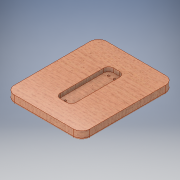
# Autodesk Inventor part: Stand
Saved by Autodesk Inventor 2017 (Build 210142000, 142)
## iProperties
Created: 2018-11-02
Part Number: Stand
Material: Wood (Oak)
Document SubType Name: Modeling
Designer: 623516
Density: 0.76 g/cm^3
Appearance: White Oak - Natural Medium Gloss
Author: 623516
Autodesk Inventor part; units mm, degrees
ref_plane "YZ Plane" through (0, 0, 0) normal (1, 0, 0) x (0, 1, 0)
ref_plane "XZ Plane" through (0, 0, 0) normal (0, 1, 0) x (-1, 0, 0)
ref_plane "XY Plane" through (0, 0, 0) normal (0, 0, 1) x (1, 0, 0)
sketch "Sketch1" plane through (0, 0, 0) normal (0, 1, 0) x (-1, 0, 0)
  line L0 (0, 0) -> (180, 0)
  line L1 (180, 0) -> (180, -220)
  line L2 (180, -220) -> (0, -220)
  line L3 (0, -220) -> (0, 0)
  line L4 (90, 0) -> (90, -220) construction
  line L5 (90, -110) -> (90, -161.5) construction
  line L6 (90, -110) -> (90, -58.5) construction
  line L7 (90, -161.5) -> (83, -161.5) construction
  line L8 (83, -161.5) -> (83, -193.1088) construction
  circle A0 centre (83, -161.5) radius 2.5
  line L9 (90, -161.5) -> (97, -161.5) construction
  circle A1 centre (97, -161.5) radius 2.5
  line L10 (90, -58.5) -> (83, -58.5) construction
  line L11 (83, -58.5) -> (83, 21.6306) construction
  circle A2 centre (83, -58.5) radius 2.5
  line L12 (90, -58.5) -> (97, -58.5) construction
  circle A3 centre (97, -58.5) radius 2.5 construction
  circle A4 centre (97, -58.5) radius 2.5
  dimension "d0" = 180
  dimension "d1" = 220
  dimension "d2" = 51.5
  dimension "d3" = 51.5
  dimension "d4" = 7
  dimension "d5" = 5
  dimension "d6" = 7
  dimension "d7" = 5
  dimension "d8" = 7
  dimension "d9" = 5
  dimension "d10" = 7
  dimension "d11" = 5
  dimension "d12" = 5
  constraints: 26 end point, 5 centre point, 5 coincident, 5 perpendicular, 3 horizontal, 3 midpoint, 2 parallel, 2 point on line
  measures "d0" distance of L1.end L2.end
  measures "d1" distance of L0.end L1.end
  measures "d2" distance of L5.start L5.end
  measures "d3" distance of L5.start L6.end
  measures "d4" distance of L5.end L7.end
  measures "d5" diameter of A0
  measures "d6" distance of L5.end L9.end
  measures "d7" diameter of A1
  measures "d8" distance of L6.end L10.end
  measures "d9" diameter of A2
  measures "d10" distance of L6.end L12.end
  measures "d11" diameter of A3
  measures "d12" diameter of A4
extrude "Extrusion1" add sketch "Sketch1" along normal blind 20
fillet "Fillet1" radius 20 4 edges at (0, 10, -220) (0, 10, 0) (-180, 10, -220) (-180, 10, 0)
sketch "Sketch2" plane through (0, 20, 0) normal (0, 1, 0) x (1, 0, 0)
  line L0 (-109, 173.5) -> (-71, 173.5)
  line L1 (-71, 173.5) -> (-71, 46.5)
  line L2 (-71, 46.5) -> (-109, 46.5)
  line L3 (-109, 46.5) -> (-109, 173.5)
  line L4 (0, 20) -> (0, 200) projected
  line L5 (-20, 220) -> (-160, 220) projected
  point P0 (0, 0)
  point P1 (-71, 110)
  point P2 (0, 110)
  point P3 (-90, 173.5)
  point P4 (-90, 220)
  dimension "d16" = 38
  dimension "d17" = 127
  constraints: 8 end point, 4 midpoint, 2 parallel, 1 horizontal, 1 horizontal alignment, 1 perpendicular, 1 vertical alignment
  measures "d16" distance of L1.end L2.end
  measures "d17" distance of L0.end L1.end
extrude "Extrusion2" cut sketch "Sketch2" against normal blind 10
fillet "Fillet2" radius 12 4 edges at (-109, 15, -173.5) (-71, 15, -173.5) (-109, 15, -46.5) (-71, 15, -46.5)
fillet "Fillet4" radius 5 8 edges at (-174.1421, 0, -214.1421) (-90, 0, -220) (-5.8579, 0, -214.1421) (0, 0, -110) (-5.8579, 0, -5.8579) (-90, 0, 0) (-174.1421, 0, -5.8579) (-180, 0, -110)
body "Solid1"
